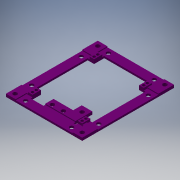
# Autodesk Inventor part: Side
Saved by Autodesk Inventor 2016 (Build 200138000, 138)
## iProperties
Created: 2015-03-28
Part Number: Side
Material: PC/ABS Plastic
Document SubType Name: Modeling
Designer: Erin
Density: 0.357273 g/cm^3
Appearance: Smooth - Purple
Mass: 3.07089 g
Surface Area: 62.8323 cm^2
Volume: 5.58344 cm^3
Author: Erin
Autodesk Inventor part; units mm, degrees
ref_plane "YZ Plane" through (0, 0, 0) normal (1, 0, 0) x (0, 1, 0)
ref_plane "XZ Plane" through (0, 0, 0) normal (0, 1, 0) x (-1, 0, 0)
ref_plane "XY Plane" through (0, 0, 0) normal (0, 0, 1) x (1, 0, 0)
sketch "Block1" plane through (0, 0, 0) normal (0, 0, 1) x (1, 0, 0)
  circle A0 centre (-3.2722, 18.9) radius 2.25
  circle A1 centre (-12.45, 7.7) radius 2.25
  circle A2 centre (-12.45, -4.3) radius 2.25
  line L0 (-6.45, -9) -> (-15.45, -9)
  line L1 (-6.45, -9) -> (-6.45, 12.4)
  line L2 (-6.45, 12.4) -> (2.9056, 12.4)
  line L3 (2.9056, 23.9) -> (-15.45, 23.9)
  line L4 (-15.45, -9) -> (-15.45, 23.9)
  line L5 (2.9056, 12.4) -> (2.9056, 23.9)
  line L6 (-6.45, 1.7) -> (-15.45, 1.7) construction
  point P0 (-7.0963, 8.6833)
  dimension "d131" = 6
  dimension "d132" = 6
  measures "d131" distance from line of A2.centre L6
  measures "d132" distance from line of A1.centre L6
sketch "Sketch1" plane through (0, 0, 0) normal (0, 0, 1) x (1, 0, 0)
  line L0 (-41.5, 50) -> (41.5, 50)
  line L1 (41.5, 50) -> (41.5, -50)
  line L2 (41.5, -50) -> (-41.5, -50)
  line L3 (-41.5, -50) -> (-41.5, 50)
  line L4 (31.5, 40) -> (-31.5, 40)
  line L5 (-31.5, 40) -> (-31.5, -40)
  line L6 (-31.5, -40) -> (31.5, -40)
  line L7 (31.5, -40) -> (31.5, 40)
  line L8 (-41.5, -45) -> (41.5, -45) construction
  line L9 (0, 71.7466) -> (0, -78.0681) construction
  line L10 (-60.2597, 0) -> (74.2823, 0) construction
  line L11 (-36.5, 50) -> (-36.5, -50) construction
  circle A0 centre (-36.5, -27) radius 2.25
  line L12 (-41.5, 45) -> (41.5, 45) construction
  circle A1 centre (-36.5, 45) radius 2.25
  circle A2 centre (-36.5, -45) radius 2.25
  circle A3 centre (-36.5, 27) radius 2.25
  circle A4 centre (-25, -45) radius 2.25
  circle A5 centre (25, -45) radius 2.25
  line L13 (30, 50) -> (30, -50) construction
  line L14 (-30, 50) -> (-30, -50) construction
  line L15 (-31, -38) -> (31, -38)
  line L16 (31, -38) -> (31, -52)
  line L17 (31, -52) -> (-31, -52)
  line L18 (-31, -52) -> (-31, -38)
  line L19 (-43.5, 33) -> (-29.5, 33)
  line L20 (-29.5, 33) -> (-29.5, -33)
  line L21 (-29.5, -33) -> (-43.5, -33)
  line L22 (-43.5, -33) -> (-43.5, 33)
  line L23 (-31.5, 40) -> (-24.5, 40)
  line L24 (-24.5, 40) -> (-24.5, 29)
  line L25 (-24.5, 29) -> (-31.5, 29)
  line L26 (-31.5, 29) -> (-31.5, 40)
  line L27 (-24.5, 29) -> (-29.5, 29)
  line L28 (-29.5, 29) -> (-29.5, 38)
  line L29 (-29.5, 38) -> (-24.5, 38)
  line L30 (-24.5, 38) -> (-24.5, 29)
  circle A6 centre (-27, 35.5) radius 1.5
  circle A7 centre (-27, 31.5) radius 1.5
  line L31 (-10.7, -38) -> (22.2, -38)
  line L32 (22.2, -38) -> (22.2, -40)
  line L33 (22.2, -40) -> (-10.7, -40)
  line L34 (-10.7, -40) -> (-10.7, -38)
  circle A8 centre (17.2, -25.8222) radius 2.25
  circle A9 centre (6, -35) radius 2.25
  circle A10 centre (-6, -35) radius 2.25
  line L35 (-10.7, -29) -> (-10.7, -38)
  line L36 (-10.7, -29) -> (10.7, -29)
  line L37 (10.7, -29) -> (10.7, -19.6444)
  line L38 (22.2, -19.6444) -> (22.2, -38)
  line L39 (-10.7, -38) -> (22.2, -38)
  line L40 (10.7, -19.6444) -> (22.2, -19.6444)
  line L41 (0, -29) -> (0, -38) construction
  point P0 (0, 0)
  point P1 (0, 50)
  point P2 (41.5, 0)
  point P3 (0, 45)
  point P4 (-27, 38)
  point P5 (-27, 29)
  dimension "d0" = 83
  dimension "d1" = 100
  dimension "d5" = 5
  dimension "d6" = 5
  dimension "d9" = 5
  dimension "d12" = 4.5
  dimension "d17" = 5
  dimension "d41" = 4.5
  dimension "d42" = 4.5
  dimension "d87" = 4.5
  dimension "d89" = 4.5
  dimension "d90" = 4.5
  dimension "d91" = 30
  dimension "d92" = 30
  dimension "d93" = 5
  dimension "d94" = 5
  dimension "d97" = 1
  dimension "d98" = 2
  dimension "d99" = 2
  dimension "d100" = 1
  dimension "d115" = 6
  dimension "d116" = 2
  dimension "d117" = 2
  dimension "d118" = 6
  dimension "d121" = 27
  dimension "d122" = 27
  dimension "d133" = 2
  dimension "d146" = 2
  dimension "d147" = 2
  dimension "d148" = 3
  dimension "d149" = 3
  dimension "d150" = 2.5
  dimension "d151" = 2.5
  dimension "d152" = 9
  dimension "d153" = 5
  constraints: 70 end point, 19 point on line, 14 parallel, 14 perpendicular, 8 centre point, 7 horizontal, 5 midpoint, 3 vertical alignment, 2 vertical, 1 horizontal alignment, 4 other
  measures "d0" distance of L1.end L2.end
  measures "d1" distance of L0.end L1.end
  measures "d5" distance between parallel lines of L8 L2
  measures "d6" distance between parallel lines of L6 L8
  measures "d9" distance between parallel lines of L11 L3
  measures "d12" diameter of A0
  measures "d17" distance between parallel lines of L12 L0
  measures "d41" diameter of A1
  measures "d42" diameter of A2
  measures "d87" diameter of A3
  measures "d89" diameter of A4
  measures "d90" diameter of A5
  measures "d91" distance between parallel lines of L13 L9
  measures "d92" distance between parallel lines of L14 L9
  measures "d93" distance from line of A4.centre L14
  measures "d94" distance from line of A5.centre L13
  measures "d97" distance between parallel lines of L14 L18
  measures "d98" distance between parallel lines of L2 L17
  measures "d99" distance between parallel lines of L6 L15
  measures "d100" distance between parallel lines of L13 L16
  measures "d115" distance from line of A0.centre L21
  measures "d116" distance between parallel lines of L5 L20
  measures "d117" distance between parallel lines of L3 L22
  measures "d118" distance from line of A3.centre L19
  measures "d121" distance from line of A0.centre L10
  measures "d122" distance from line of A3.centre L10
  measures "d146" distance between parallel lines of L29 L4
  measures "d147" distance between parallel lines of L5 L28
  measures "d148" diameter of A6
  measures "d149" diameter of A7
  measures "d150" distance from line of A6.centre L29
  measures "d151" distance from line of A7.centre L25
  measures "d152" distance of L29.end L24.end
  measures "d153" distance of L28.end L29.end
extrude "Extrusion1" add sketch "Sketch1" against normal blind 3 contours L0 L1 L2 L16 L6 L7 L4 L5 L19 L3 | L19 L5 L21 L3 | L21 L5 L6 L18 L2 L3 | L2 L18 L6 L16 | A0 | A1 | A2 | A3 | A4 | A5
extrude "Extrusion2" cut sketch "Sketch1" against normal blind 10 contours A0 | A1 | A2 | A3
mirror "Mirror1" about plane through (0, 0, 0) normal (1, 0, 0) of "Extrusion2"
extrude "Extrusion8" cut sketch "Sketch1" against normal blind 10 contours A4 | A5
extrude "Extrusion17" add sketch "Sketch1" against normal blind 3 contours L6 L34 L15 L32
extrude "Extrusion9" cut sketch "Sketch1" against normal blind 1 contours L16 L17 L18 L2 | L2 L18 L6 L16 | L6 L32 L15 L16 | L18 L15 L34 L6 | L6 L34 L15 L32
extrude "Extrusion14" add sketch "Sketch1" against normal blind 3 contours L19 L20 L25 L5 | L5 L4 L24 L29 L28 L19
extrude "Extrusion11" cut sketch "Sketch1" against normal blind 1 contours L19 L5 L21 L3 | L3 L21 L22 L19 | L19 L20 L25 L5 | L5 L25 L20 L21
mirror "Mirror4" about plane through (0, 0, 0) normal (0, 1, 0) of "Extrusion8", "Extrusion9"
mirror "Mirror5" about plane through (0, 0, 0) normal (1, 0, 0) of "Extrusion11"
extrude "Extrusion13" add sketch "Sketch1" against normal blind 3 contours L15 L35 L36 L37 L40 L38
extrude "Extrusion15" add sketch "Sketch1" against normal blind 3 contours L28 L29 L24 L25 L20
extrude "Extrusion16" add sketch "Sketch1" along normal blind 1.5 contours L28 L29 L24 L25 L20
mirror "Mirror6" about plane through (0, 0, 0) normal (1, 0, 0) of "Extrusion15", "Extrusion16", "Extrusion14"
mirror "Mirror7" about plane through (0, 0, 0) normal (0, 1, 0) of "Extrusion15", "Extrusion16", "Extrusion14", "Mirror6"
extrude "Extrusion18" cut sketch "Sketch1" against normal blind 1 contours L16 L17 L18 L2 | L2 L18 L6 L16 | L6 L32 L15 L16 | L18 L15 L34 L6
extrude "Extrusion19" cut sketch "Sketch1" against normal blind 1 contours L19 L5 L21 L3 | L3 L21 L22 L19 | L19 L20 L25 L5 | L5 L25 L20 L21
mirror "Mirror8" about plane through (0, 0, 0) normal (1, 0, 0) of "Extrusion19"
equation "\"d12\" = screw"
equation "\"d41\" = screw"
equation "\"d42\" = screw"
equation "\"d87\" = screw"
equation "\"d89\" = screw"
equation "\"d90\" = screw"
equation "\"d37\" = mat"
equation "\"screw\" = 4.5"
equation "\"mat\" = 3"
body "Solid1"
